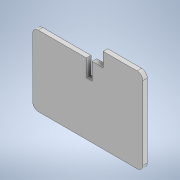
# Autodesk Inventor part: pcb_balun_bottom
Saved by Autodesk Inventor 2020.2 (Build 242310000, 310)
## iProperties
Created: 2020-09-26
Part Number: pcb_balun_bottom
Material: Generic
Document SubType Name: Modeling
Designer: Krishna Makhija
Density: 1 g/cm^3
Appearance: Default
Author: Krishna Makhija
Autodesk Inventor part; units mm, degrees
ref_plane "YZ Plane" through (0, 0, 0) normal (1, 0, 0) x (0, 1, 0)
ref_plane "XZ Plane" through (0, 0, 0) normal (0, 1, 0) x (-1, 0, 0)
ref_plane "XY Plane" through (0, 0, 0) normal (0, 0, 1) x (1, 0, 0)
sketch "Sketch5" plane through (0, 0, 0) normal (0, 0, 1) x (1, 0, 0)
  line L0 (19.5002, -12.5002) -> (-19.5002, -12.5002)
  line L1 (-19.5002, -12.5002) -> (-19.5002, 12.5002)
  line L2 (19.5002, 12.5002) -> (19.5002, -12.5002)
  line L3 (19.5002, -12.5002) -> (-19.5002, 12.5002) construction
  line L4 (-19.5002, -12.5002) -> (19.5002, 12.5002) construction
  line L5 (1.6, 6.4998) -> (-0.4, 6.4998)
  line L6 (-0.4, 6.4998) -> (-0.4, 12.5002)
  line L7 (1.6, 12.5002) -> (1.6, 6.4998)
  line L8 (1.6, 6.4998) -> (-0.4, 12.5002) construction
  line L9 (-0.4, 6.4998) -> (1.6, 12.5002) construction
  line L10 (5.4998, 12.5002) -> (5.4998, 17.5003)
  line L11 (5.4998, 17.5003) -> (19.5002, 17.5003)
  line L12 (19.5002, 17.5003) -> (19.5002, 12.5002)
  line L13 (-19.5002, 12.5002) -> (-0.4, 12.5002)
  line L14 (1.6, 12.5002) -> (5.4998, 12.5002)
  constraints: 30 end point, 3 horizontal, 3 parallel, 2 perpendicular, 1 collinear
extrude "Extrusion4" add sketch "Sketch5" along normal blind 1.6
fillet "Fillet4" radius 2 4 edges at (19.5002, 17.5003, 0.8) (-19.5002, 12.5002, 0.8) (19.5002, -12.5002, 0.8) (-19.5002, -12.5002, 0.8)
body "Solid4"
